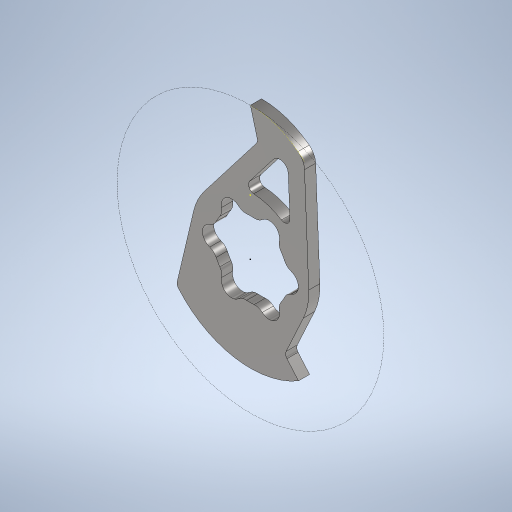
# Autodesk Inventor part: Blade
Saved by Autodesk Inventor 2023.4 (Build 274418000, 418)
## iProperties
Created: 2023-11-12
Part Number: Blade
Material: Steel, Alloy
Document SubType Name: Modeling
Designer: Nathan Cai
Density: 7.73 g/cm^3
Appearance: Semi-Polished
Mass: 213.362 g
Surface Area: 125.78 cm^2
Volume: 27.6019 cm^3
Author: Nathan Cai
Autodesk Inventor part; units mm, degrees
ref_plane "YZ Plane" through (0, 0, 0) normal (1, 0, 0) x (0, 1, 0)
ref_plane "XZ Plane" through (0, 0, 0) normal (0, 1, 0) x (-1, 0, 0)
ref_plane "XY Plane" through (0, 0, 0) normal (0, 0, 1) x (1, 0, 0)
sketch "Sketch1" plane through (0, 0, 0) normal (0, 0, 1) x (1, 0, 0)
  circle A0 centre (0, 0) radius 76.2 construction
  circle A1 centre (0, 0) radius 21.5
  circle A2 centre (0, 0) radius 21.5 construction
  circle A3 centre (0, 0) radius 33.3375
  line L0 (0, 76.2) -> (0, 0) construction
  line L1 (0, 76.2) -> (4.2947, 60.1719)
  line L2 (4.2947, 60.1719) -> (-26.4022, 20.3547)
  circle A4 centre (0, 0) radius 60.325 construction
  arc A5 (30.7227, 63.8735) -> (0, 76.2) centre (0, 31.75) ccw
  line L3 (30.7227, 63.8735) -> (33.309, 1.3784)
  circle A6 centre (0, 0) radius 53.975 construction
  line L4 (27.435, -46.4825) -> (0, 0) construction
  line L5 (27.435, -46.4825) -> (19.5403, -37.2553)
  line L6 (19.5403, -37.2553) -> (30.278, -13.951)
  circle A7 centre (0, 0) radius 42.0688 construction
  arc A8 (-42.2119, -33.6371) -> (27.435, -46.4825) centre (0, 0) ccw
  line L7 (-42.2119, -33.6371) -> (-32.4426, 7.6724)
  line L8 (-42.2119, -33.6371) -> (0, 0) construction
  line L9 (-4.6134, 33.0167) -> (13.0978, 55.9902)
  line L10 (22.8274, 24.296) -> (21.628, 53.2793)
  arc A9 (21.628, 53.2793) -> (13.0978, 55.9902) centre (16.8696, 53.0824) ccw
  line L11 (0, 0) -> (-10.75, 18.6195) construction
  arc A10 (-6.7508, 22.9574) -> (-16.5062, 17.3251) centre (-10.75, 18.6195) ccw
  arc A11 (-17.4815, 12.5159) -> (-16.5062, 17.3251) centre (-22.3601, 16.0087) ccw
  arc A12 (-6.7508, 22.9574) -> (-2.0983, 21.3974) centre (-2.6839, 27.3687) ccw
  arc A13 (16.5062, 17.3251) -> (17.4815, 12.5159) centre (22.3601, 16.0087) ccw
  arc A14 (16.5062, 17.3251) -> (6.7508, 22.9574) centre (10.75, 18.6195) ccw
  arc A15 (2.0983, 21.3974) -> (6.7508, 22.9574) centre (2.6839, 27.3687) ccw
  arc A16 (23.2571, -5.6323) -> (19.5798, -8.8815) centre (25.044, -11.36) ccw
  arc A17 (23.2571, -5.6323) -> (23.2571, 5.6323) centre (21.5, 0) ccw
  arc A18 (19.5798, 8.8815) -> (23.2571, 5.6323) centre (25.044, 11.36) ccw
  arc A19 (6.7508, -22.9574) -> (2.0983, -21.3974) centre (2.6839, -27.3687) ccw
  arc A20 (6.7508, -22.9574) -> (16.5062, -17.3251) centre (10.75, -18.6195) ccw
  arc A21 (17.4815, -12.5159) -> (16.5062, -17.3251) centre (22.3601, -16.0087) ccw
  arc A22 (-16.5062, -17.3251) -> (-17.4815, -12.5159) centre (-22.3601, -16.0087) ccw
  arc A23 (-16.5062, -17.3251) -> (-6.7508, -22.9574) centre (-10.75, -18.6195) ccw
  arc A24 (-2.0983, -21.3974) -> (-6.7508, -22.9574) centre (-2.6839, -27.3687) ccw
  arc A25 (-23.2571, 5.6323) -> (-19.5798, 8.8815) centre (-25.044, 11.36) ccw
  arc A26 (-23.2571, 5.6323) -> (-23.2571, -5.6323) centre (-21.5, 0) ccw
  arc A27 (-19.5798, -8.8815) -> (-23.2571, -5.6323) centre (-25.044, -11.36) ccw
  point P0 (25.3939, -0.9713)
  point P1 (-23.0466, 22.3171)
  point P2 (-2.0983, 21.3974)
  point P3 (2.0983, 21.3974)
  point P4 (17.4815, 12.5159)
  point P5 (19.5798, -8.8815)
  point P6 (2.0983, -21.3974)
  point P7 (-2.0983, -21.3974)
  point P8 (-17.4815, -12.5159)
  point P9 (-19.5798, -8.8815)
  point P10 (-19.5798, 8.8815)
  dimension "d0" = 152.4
  dimension "d14" = 15.875
  dimension "d17" = 84.1375
  dimension "d1" = 43
  dimension "d2" = 43
  dimension "d8" = 66.675
  dimension "d9" = 15
  dimension "d11" = 44.45
  dimension "d12" = 40
  dimension "d15" = 107.95
  dimension "d16" = 10
  dimension "d18" = 30.55
  dimension "d19" = 82
  dimension "d28" = 9.525
  dimension "d29" = 9.525
  dimension "d30" = 4.7625
  dimension "d46" = 11.8
  dimension "d47" = 6
  dimension "d48" = 30
  dimension "d51" = 360
  constraints: 52 point on circle, 25 centre point, 24 end point, 8 coincident, 8 tangent, 3 symmetric about line, 2 concentric, 2 parallel, 1 vertical, 1 vertical alignment, 71 other
  measures "d1" diameter of A1
  measures "d2" diameter of A2
  measures "d8" diameter of A3
  measures "d9" angle of L0 L1
  measures "d11" radius of A5
  measures "d12" angle of L2 L3
  measures "d15" diameter of A6
  measures "d16" angle of L4 L5
  measures "d18" angle of L0 L4
  measures "d19" angle of L4 L8
  measures "d28" distance between parallel lines of L3 L10
  measures "d29" distance between parallel lines of L2 L9
  measures "d30" radius of A9
  measures "d46" diameter of A10
  measures "d47" radius of A11
  measures "d48" angle of L0 L11
extrude "Extrusion1" add sketch "Sketch1" along normal blind 6.35 contours A3 | A3 L10 A9 L9 L2 L1 A5 L3 | L6 L5 A8 L7 A3
fillet "Fillet1" radius 3.175 4 edges at (19.5403, -37.2553, 3.175) (4.2947, 60.1719, 3.175) (-4.6134, 33.0167, 3.175) (22.8274, 24.296, 3.175)
fillet "Fillet3" radius 3.175 1 edges at (-42.2119, -33.6371, 3.175)
sketch "Sketch2" plane through (0, 0, 6.35) normal (0, 0, 1) x (1, 0, 0)
  arc A0 (30.7227, 63.8735) -> (0, 76.2) centre (0, 31.75) ccw construction
  circle A1 centre (0, 0) radius 76.2 construction
  constraints: 1 coincident, 1 vertical alignment, 2 other
fillet "Fillet4" radius 9.525 1 edges at (30.7227, 63.8735, 3.175)
equation "\"d29\" = d28"
body "Solid1"
